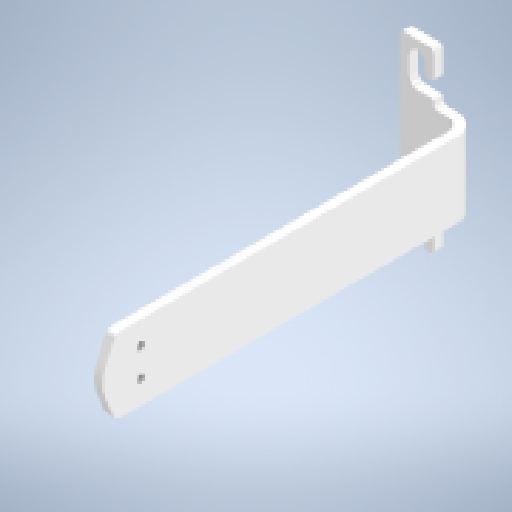
# Autodesk Inventor part: Spool Holder Left
Saved by Autodesk Inventor 2024 (Build 280153000, 153)
## iProperties
Created: 2025-01-02
Part Number: Spool Holder Left
Material: Aluminum 6061
Document SubType Name: Sheet Metal
Designer: Ishaan
Density: 2.7 g/cm^3
Sheet Metal Rule: SendCutSend_3-16_Alu
Appearance: Aluminum - Flat
Author: Ishaan
Autodesk Inventor part; units mm, degrees
ref_plane "YZ Plane" through (0, 0, 0) normal (1, 0, 0) x (0, 1, 0)
ref_plane "XZ Plane" through (0, 0, 0) normal (0, 1, 0) x (-1, 0, 0)
ref_plane "XY Plane" through (0, 0, 0) normal (0, 0, 1) x (1, 0, 0)
sketch "Sketch3" plane through (0, 0, 0) normal (0, 0, 1) x (1, 0, 0)
  line L0 (9, -47.5) -> (-9, -47.5)
  line L1 (-9, -47.5) -> (-9, 47.5)
  line L2 (-9, 47.5) -> (9, 47.5)
  line L3 (9, 47.5) -> (9, -47.5)
  line L4 (9, -47.5) -> (-9, 47.5) construction
  line L5 (-9, -47.5) -> (9, 47.5) construction
  line L6 (9, 47.5) -> (14, 47.5)
  line L7 (14, 47.5) -> (14, -47.5)
  line L8 (14, -47.5) -> (9, -47.5)
  line L9 (9, -47.5) -> (9, 47.5)
  point P0 (0, 0)
  dimension "d10" = 18
  dimension "d11" = 95
  dimension "d25" = 5
  measures "d10" distance of L1.end L2.end
  measures "d11" distance of L0.end L1.end
  measures "d25" distance of L7.end L8.end
extrude "Plate2" add sketch "Sketch3" along normal blind 4.7625 contours L0 L1 L2 L3
sketch "Sketch4" plane through (0, 0, 4.7625) normal (0, 0, 1) x (1, 0, 0)
  line L0 (-9, -47.5) -> (-9, 47.5) construction
  line L1 (0, 28.5) -> (0, 38.5) construction
  line L2 (4.2, 28.5) -> (4.2, 38.5)
  line L3 (-4.2, 38.5) -> (-4.2, 28.5)
  arc A0 (-4.2, 28.5) -> (4.2, 28.5) centre (0, 28.5) ccw
  arc A1 (4.2, 38.5) -> (-4.2, 38.5) centre (0, 38.5) ccw
  line L4 (0, -35.5) -> (0, -47.5) construction
  line L5 (-9, -47.5) -> (9, -47.5) projected
  line L6 (-4.2, -35.5) -> (-4.2, -47.5)
  line L7 (4.2, -47.5) -> (4.2, -35.5)
  arc A2 (4.2, -35.5) -> (-4.2, -35.5) centre (0, -35.5) ccw
  arc A3 (-4.2, -47.5) -> (4.2, -47.5) centre (0, -47.5) ccw
  line L8 (0, -41) -> (0, -35.5) construction
  line L9 (0, 28.5) -> (9, 28.5) construction
  line L10 (0, 32.7) -> (9, 32.7)
  line L11 (9, 24.3) -> (0, 24.3)
  arc A4 (0, 32.7) -> (0, 24.3) centre (0, 28.5) ccw
  arc A5 (9, 24.3) -> (9, 32.7) centre (9, 28.5) ccw
  line L12 (9, 47.5) -> (9, -47.5) projected
  line L13 (-9, 47.5) -> (9, 47.5) projected
  point P0 (0, 0)
  point P1 (0, 33.5)
  point P2 (0, -41.5)
  point P3 (4.5, 28.5)
  point P4 (0, 42.7)
  point P5 (4.2, 32.7)
  point P6 (0, 24.3)
  dimension "d15" = 10
  dimension "d61" = 4.2
  dimension "d62" = 12
  dimension "d63" = 4.8
  dimension "d64" = 4.8
  constraints: 26 end point, 13 point on circle, 13 tangent, 6 centre point, 4 midpoint, 4 point on line, 3 parallel, 2 vertical, 1 collinear, 1 equal radius, 1 vertical alignment
  measures "d15" distance of L1.start L1.end
  measures "d61" radius of A0
  measures "d62" distance of L4.start L4.end
  measures "d63" distance between parallel lines of L0 L3
  measures "d64" distance from line of point (0, 42.7) L13
extrude "Extrusion2" cut sketch "Sketch4" against normal through all contours A0 A4 L10 L2 | L2 L10 L12 L11 A0 | L10 A4 L3 A1 L2 | L6 A2 L7 L5
fillet "Fillet3" radius 1 5 edges at (-4.2, -47.5, 2.3813) (4.2, -47.5, 2.3813) (9, 32.7, 2.3813) (9, 24.3, 2.3813) (4.2, 32.7, 2.3813)
fillet "Fillet4" radius 2 4 edges at (-9, 47.5, 2.3813) (-9, -47.5, 2.3813) (9, 47.5, 2.3813) (9, -47.5, 2.3813)
sketch "Sketch5" plane through (0, 0, 4.7625) normal (0, 0, 1) x (1, 0, 0)
  line L0 (16.8875, -20) -> (9, -20)
  line L1 (9, -20) -> (9, 20)
  line L2 (9, 20) -> (16.8875, 20)
  line L3 (16.8875, 20) -> (16.8875, -20)
  line L4 (16.8875, -20) -> (9, 20) construction
  line L5 (9, -20) -> (16.8875, 20) construction
  line L6 (28, 20.7219) -> (28, -16.4847) construction
  line L7 (9, 24.3) -> (9, -47.5) projected
  point P0 (0, 0)
  point P1 (12.9438, 0)
  point P2 (14, -29.8149)
  dimension "d20" = 40
  dimension "d21" = 28
  dimension "d22" = 11.1125
  constraints: 14 end point, 2 midpoint, 2 parallel, 1 collinear, 1 horizontal, 1 horizontal alignment, 1 perpendicular, 1 vertical
  measures "d20" distance of L0.end L1.end
  measures "d21" distance from line of point (0, 0) L6
  measures "d22" distance between parallel lines of L6 L3
extrude "Extrusion3" add sketch "Sketch5" against normal up to surface (4.7625 mm away)
sketch "Sketch6" plane through (23.2375, 20, 11.1125) normal (1, 0, 0) x (0, 1, 0)
  line L0 (-40, 0) -> (0, 0)
  line L1 (0, 0) -> (0, 173.65)
  line L2 (0, 173.65) -> (-40, 173.65)
  line L3 (-40, 173.65) -> (-40, 0)
  constraints: 6 end point, 1 horizontal, 1 perpendicular, 1 vertical
edge flange "Flange1" height 180 angle 90 thickness 4.7625 bend radius 6.35 thickness toward (1, 0, 0) relief tear relief width 4.7625 relief depth 2.3813 edges at (16.8875, 0, 4.7625) wall of the first edge with corners at (23.2375, -20, 11.1125) (23.2375, 20, 11.1125) (23.2375, 20, 184.7625) (23.2375, -20, 184.7625)
bend "Bend1"
corner "Corner1"
sketch "Sketch7" plane through (23.2375, -20, 184.7625) normal (-1, 0, 0) x (0, 0, 1)
  line L0 (-173.65, 40) -> (-173.65, 0) construction
  line L1 (0, 0) -> (-173.65, 0) construction
  line L2 (0, 0) -> (0, 40) projected
  line L3 (0, 40) -> (-173.65, 40) construction
  line L4 (0, 40) -> (13.3636, 40)
  line L5 (13.3636, 40) -> (18.4776, 27.6537)
  line L6 (18.4776, 12.3463) -> (13.3636, 0)
  line L7 (13.3636, 0) -> (0, 0)
  line L8 (0, 0) -> (0, 40) construction
  circle A0 centre (0, 20) radius 17 construction
  arc A1 (18.4776, 12.3463) -> (18.4776, 27.6537) centre (0, 20) ccw
  line L9 (0, 27.5) -> (0, 12.5) construction
  line L10 (0, 0) -> (0, 40) construction
  circle A2 centre (0, 27.5) radius 5 construction
  circle A3 centre (0, 12.5) radius 5 construction
  circle A4 centre (0, 20) radius 15 construction
  point P0 (-184.7625, 20)
  point P1 (21.6478, 20)
  dimension "d36" = 135
  dimension "d44" = 3
  dimension "d45" = 3
  dimension "d49" = 15
  dimension "d50" = 10
  dimension "d51" = 10
  dimension "d59" = 30
  constraints: 12 end point, 5 centre point, 4 coincident, 4 midpoint, 2 point on circle, 2 point on line, 2 tangent, 1 concentric, 1 horizontal, 1 horizontal alignment, 1 parallel, 1 perpendicular, 1 vertical, 1 vertical alignment
  measures "d36" angle of L6 L5
  measures "d44" distance edge to line of A0 L4
  measures "d45" radial gap between concentric circles of A0 A1
  measures "d49" distance of L9.start L9.end
  measures "d50" diameter of A2
  measures "d51" diameter of A3
  measures "d59" diameter of A4
extrude "Extrusion4" add sketch "Sketch7" against normal up to surface (4.7625 mm away)
fillet "Fillet7" radius 5 2 edges at (25.6188, 20, 198.1261) (25.6188, -20, 198.1261)
fillet "Fillet8" radius 2 2 edges at (9, 20, 2.3813) (9, -20, 2.3813)
hole "Hole1" at (23.2375, 7.5, 184.7625) at (23.2375, -7.5, 184.7625) direction (1, 0, 0) diameter 4.134 end through all thread size "M5x0.8" class "6H" standard "ANSI Metric M Profile"
equation "\"d64\" = d63"
equation "\"d45\" = d44"
equation "\"d57\" = Thickness"
equation "\"d7\" = Thickness"
equation "\"d26\" = BendReliefWidth"
equation "\"d27\" = BendReliefDepth"
equation "\"d28\" = MinimumRemnant"
equation "\"d29\" = TransitionRadius"
equation "\"d32\" = BendRadius"
equation "\"d33\" = CornerReliefSize"
equation "\"d34\" = GapSize"
equation "\"d35\" = JacobiRadiusSize"
equation "\"BendReliefWidth\" = Thickness"
equation "\"BendReliefDepth\" = 0.5 * Thickness"
equation "\"CornerReliefSize\" = 4 * Thickness"
equation "\"MinimumRemnant\" = 2 * Thickness"
equation "\"TransitionRadius\" = BendRadius"
equation "\"JacobiRadiusSize\" = BendRadius"
equation "\"GapSize\" = Thickness"
equation "\"Thickness\" = 4.7625"
equation "\"BendRadius\" = 6.35"
body "Solid2"
